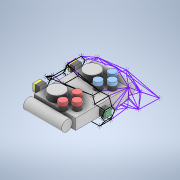
# Autodesk Inventor part: Obudowa_v1
Saved by Autodesk Inventor 2020 (Build 240168000, 168)
## iProperties
Created: 2020-04-14
Part Number: Obudowa_v1
Material: Generic
Document SubType Name: Modeling
Designer: atmat
Density: 1 g/cm^3
Appearance: Default
Author: atmat
Autodesk Inventor part; units mm, degrees
ref_plane "XY Plane" through (0, 0, 0) normal (0, 0, 1) x (1, 0, 0)
sketch "Sketch1" plane through (0, 0, 0) normal (0, 1, 0) x (-1, 0, 0)
  line L0 (35.245, 45.085) -> (-35.245, 45.085)
  line L1 (-35.245, 45.085) -> (-35.245, -45.085)
  line L2 (-35.245, -45.085) -> (35.245, -45.085)
  line L3 (35.245, -45.085) -> (35.245, 45.085)
  circle A0 centre (11.745, 29.845) radius 13
  circle A1 centre (11.745, -29.845) radius 13
  line L4 (-10.475, 45.085) -> (-10.475, -45.085) construction
  circle A2 centre (-10.475, 41.905) radius 6.5
  circle A3 centre (-10.475, 17.775) radius 6.5
  circle A4 centre (-10.475, -17.775) radius 6.5
  circle A5 centre (-10.475, -41.905) radius 6.5
  circle A6 centre (-22.545, 29.845) radius 6.5
  circle A7 centre (-22.545, -29.845) radius 6.5
  point P0 (0, 0)
  dimension "d0" = 90.17
  dimension "d1" = 45.085
  dimension "d2" = 35.245
  dimension "d3" = 70.49
  dimension "d4" = 15.24
  dimension "d5" = 15.24
  dimension "d6" = 23.5
  dimension "d7" = 23.5
  dimension "d8" = 26
  dimension "d9" = 26
  dimension "d10" = 45.72
  dimension "d11" = 13
  dimension "d12" = 13
  dimension "d13" = 13
  dimension "d14" = 13
  dimension "d15" = 3.18
  dimension "d16" = 3.18
  dimension "d17" = 24.13
  dimension "d18" = 24.13
  dimension "d19" = 13
  dimension "d20" = 12.07
  dimension "d21" = 12.07
  dimension "d22" = 0
  dimension "d23" = 0
  dimension "d24" = 13
  constraints: 10 end point, 8 centre point, 6 point on line, 2 parallel, 2 perpendicular, 1 horizontal
  measures "d0" distance of L2.end L0.start
  measures "d1" distance from line of point (0, 0) L0
  measures "d2" distance from line of point (0, 0) L3
  measures "d3" distance of L1.end L2.end
  measures "d4" distance from line of L0 A0.centre
  measures "d5" distance from line of L2 A1.centre
  measures "d6" distance from line of L3 A1.centre
  measures "d7" distance from line of L3 A0.centre
  measures "d8" diameter of A0
  measures "d9" diameter of A1
  measures "d10" distance between parallel lines of L3 L4
  measures "d11" diameter of A2
  measures "d12" diameter of A3
  measures "d13" diameter of A4
  measures "d14" diameter of A5
  measures "d15" distance from line of L0 A2.centre
  measures "d16" distance from line of L2 A5.centre
  measures "d17" distance of A3.centre A2.centre
  measures "d18" distance of A4.centre A5.centre
  measures "d19" diameter of A6
  measures "d20" horizontal distance of A2.centre A6.centre
  measures "d21" horizontal distance of A5.centre A7.centre
  measures "d22" vertical distance of A6.centre A0.centre
  measures "d23" vertical distance of A7.centre A1.centre
  measures "d24" diameter of A7
extrude "Extrusion1" add sketch "Sketch1" along normal blind 11 contours A0 | A1
sketch "Sketch2" plane through (0, 0, 0) normal (0, 1, 0) x (-1, 0, 0)
  line L0 (35.245, 45.085) -> (-35.245, 45.085)
  line L1 (-35.245, 45.085) -> (-35.245, -45.085)
  line L2 (-35.245, -45.085) -> (35.245, -45.085)
  line L3 (35.245, -45.085) -> (35.245, 45.085)
  circle A0 centre (11.745, 29.845) radius 13
  circle A1 centre (11.745, -29.845) radius 13
  line L4 (-10.475, 45.085) -> (-10.475, -45.085) construction
  circle A2 centre (-10.475, 41.905) radius 6.5
  circle A3 centre (-10.475, 17.775) radius 6.5
  circle A4 centre (-10.475, -17.775) radius 6.5
  circle A5 centre (-10.475, -41.905) radius 6.5
  circle A6 centre (-22.545, 29.845) radius 6.5
  circle A7 centre (-22.545, -29.845) radius 6.5
  point P0 (0, 0)
  dimension "d27" = 90.17
  dimension "d28" = 45.085
  dimension "d29" = 35.245
  dimension "d30" = 70.49
  dimension "d31" = 15.24
  dimension "d32" = 15.24
  dimension "d33" = 23.5
  dimension "d34" = 23.5
  dimension "d35" = 26
  dimension "d36" = 26
  dimension "d37" = 45.72
  dimension "d38" = 13
  dimension "d39" = 13
  dimension "d40" = 13
  dimension "d41" = 13
  dimension "d42" = 3.18
  dimension "d43" = 3.18
  dimension "d44" = 24.13
  dimension "d45" = 24.13
  dimension "d46" = 13
  dimension "d47" = 12.07
  dimension "d48" = 12.07
  dimension "d49" = 0
  dimension "d50" = 0
  dimension "d51" = 13
  constraints: 10 end point, 8 centre point, 6 point on line, 2 parallel, 2 perpendicular, 1 horizontal
  measures "d27" distance of L2.end L0.start
  measures "d28" distance from line of point (0, 0) L0
  measures "d29" distance from line of point (0, 0) L3
  measures "d30" distance of L1.end L2.end
  measures "d31" distance from line of L0 A0.centre
  measures "d32" distance from line of L2 A1.centre
  measures "d33" distance from line of L3 A1.centre
  measures "d34" distance from line of L3 A0.centre
  measures "d35" diameter of A0
  measures "d36" diameter of A1
  measures "d37" distance between parallel lines of L3 L4
  measures "d38" diameter of A2
  measures "d39" diameter of A3
  measures "d40" diameter of A4
  measures "d41" diameter of A5
  measures "d42" distance from line of L0 A2.centre
  measures "d43" distance from line of L2 A5.centre
  measures "d44" distance of A3.centre A2.centre
  measures "d45" distance of A4.centre A5.centre
  measures "d46" diameter of A6
  measures "d47" horizontal distance of A2.centre A6.centre
  measures "d48" horizontal distance of A5.centre A7.centre
  measures "d49" vertical distance of A6.centre A0.centre
  measures "d50" vertical distance of A7.centre A1.centre
  measures "d51" diameter of A7
extrude "Extrusion2" add sketch "Sketch2" along normal blind 7 contours A2 L0 | L0 A2 | A5 L2 | L2 A5 | A3 | A4 | A6 | A7
ref_plane "Work Plane1" through (0, 7, 0) normal (0, 1, 0) x (-1, 0, 0)
sketch "Sketch3" plane through (0, 7, 0) normal (0, 1, 0) x (-1, 0, 0)
  line L0 (35.245, 45.085) -> (-35.245, 45.085)
  line L1 (-35.245, 45.085) -> (-35.245, -45.085)
  line L2 (-35.245, -45.085) -> (35.245, -45.085)
  line L3 (35.245, -45.085) -> (35.245, 45.085)
  circle A0 centre (11.745, 29.845) radius 13
  circle A1 centre (11.745, -29.845) radius 13
  line L4 (-10.475, 45.085) -> (-10.475, -45.085) construction
  circle A2 centre (-10.475, 41.905) radius 6.5
  circle A3 centre (-10.475, 17.775) radius 6.5
  circle A4 centre (-10.475, -17.775) radius 6.5
  circle A5 centre (-10.475, -41.905) radius 6.5
  circle A6 centre (-22.545, 29.845) radius 6.5
  circle A7 centre (-22.545, -29.845) radius 6.5
  point P0 (0, 0)
  dimension "d55" = 90.17
  dimension "d56" = 45.085
  dimension "d57" = 35.245
  dimension "d58" = 70.49
  dimension "d59" = 15.24
  dimension "d60" = 15.24
  dimension "d61" = 23.5
  dimension "d62" = 23.5
  dimension "d63" = 26
  dimension "d64" = 26
  dimension "d65" = 45.72
  dimension "d66" = 13
  dimension "d67" = 13
  dimension "d68" = 13
  dimension "d69" = 13
  dimension "d70" = 3.18
  dimension "d71" = 3.18
  dimension "d72" = 24.13
  dimension "d73" = 24.13
  dimension "d74" = 13
  dimension "d75" = 12.07
  dimension "d76" = 12.07
  dimension "d77" = 0
  dimension "d78" = 0
  dimension "d79" = 13
  constraints: 10 end point, 8 centre point, 6 point on line, 2 parallel, 2 perpendicular, 1 horizontal
  measures "d55" distance of L2.end L0.start
  measures "d56" distance from line of point (0, 0) L0
  measures "d57" distance from line of point (0, 0) L3
  measures "d58" distance of L1.end L2.end
  measures "d59" distance from line of L0 A0.centre
  measures "d60" distance from line of L2 A1.centre
  measures "d61" distance from line of L3 A1.centre
  measures "d62" distance from line of L3 A0.centre
  measures "d63" diameter of A0
  measures "d64" diameter of A1
  measures "d65" distance between parallel lines of L3 L4
  measures "d66" diameter of A2
  measures "d67" diameter of A3
  measures "d68" diameter of A4
  measures "d69" diameter of A5
  measures "d70" distance from line of L0 A2.centre
  measures "d71" distance from line of L2 A5.centre
  measures "d72" distance of A3.centre A2.centre
  measures "d73" distance of A4.centre A5.centre
  measures "d74" diameter of A6
  measures "d75" horizontal distance of A2.centre A6.centre
  measures "d76" horizontal distance of A5.centre A7.centre
  measures "d77" vertical distance of A6.centre A0.centre
  measures "d78" vertical distance of A7.centre A1.centre
  measures "d79" diameter of A7
extrude "Extrusion3" add sketch "Sketch3" along normal blind 6 separate body contours A2 L0 | L0 A2 | A5 L2 | L2 A5 | A3 | A4 | A6 | A7
sketch "Sketch4" plane through (0, 0, 0) normal (0, 1, 0) x (-1, 0, 0)
  line L0 (35.245, 45.085) -> (-35.245, 45.085)
  line L1 (-35.245, 45.085) -> (-35.245, -45.085)
  line L2 (-35.245, -45.085) -> (35.245, -45.085)
  line L3 (35.245, -45.085) -> (35.245, 45.085)
  circle A0 centre (11.745, 29.845) radius 13
  circle A1 centre (11.745, -29.845) radius 13
  line L4 (-10.475, 45.085) -> (-10.475, -45.085) construction
  circle A2 centre (-10.475, 41.905) radius 6.5
  circle A3 centre (-10.475, 17.775) radius 6.5
  circle A4 centre (-10.475, -17.775) radius 6.5
  circle A5 centre (-10.475, -41.905) radius 6.5
  circle A6 centre (-22.545, 29.845) radius 6.5
  circle A7 centre (-22.545, -29.845) radius 6.5
  point P0 (0, 0)
  dimension "d82" = 90.17
  dimension "d83" = 45.085
  dimension "d84" = 35.245
  dimension "d85" = 70.49
  dimension "d86" = 15.24
  dimension "d87" = 15.24
  dimension "d88" = 23.5
  dimension "d89" = 23.5
  dimension "d90" = 26
  dimension "d91" = 26
  dimension "d92" = 45.72
  dimension "d93" = 13
  dimension "d94" = 13
  dimension "d95" = 13
  dimension "d96" = 13
  dimension "d97" = 3.18
  dimension "d98" = 3.18
  dimension "d99" = 24.13
  dimension "d100" = 24.13
  dimension "d101" = 13
  dimension "d102" = 12.07
  dimension "d103" = 12.07
  dimension "d104" = 0
  dimension "d105" = 0
  dimension "d106" = 13
  constraints: 10 end point, 8 centre point, 6 point on line, 2 parallel, 2 perpendicular, 1 horizontal
  measures "d82" distance of L2.end L0.start
  measures "d83" distance from line of point (0, 0) L0
  measures "d84" distance from line of point (0, 0) L3
  measures "d85" distance of L1.end L2.end
  measures "d86" distance from line of L0 A0.centre
  measures "d87" distance from line of L2 A1.centre
  measures "d88" distance from line of L3 A1.centre
  measures "d89" distance from line of L3 A0.centre
  measures "d90" diameter of A0
  measures "d91" diameter of A1
  measures "d92" distance between parallel lines of L3 L4
  measures "d93" diameter of A2
  measures "d94" diameter of A3
  measures "d95" diameter of A4
  measures "d96" diameter of A5
  measures "d97" distance from line of L0 A2.centre
  measures "d98" distance from line of L2 A5.centre
  measures "d99" distance of A3.centre A2.centre
  measures "d100" distance of A4.centre A5.centre
  measures "d101" diameter of A6
  measures "d102" horizontal distance of A2.centre A6.centre
  measures "d103" horizontal distance of A5.centre A7.centre
  measures "d104" vertical distance of A6.centre A0.centre
  measures "d105" vertical distance of A7.centre A1.centre
  measures "d106" diameter of A7
extrude "Extrusion4" add sketch "Sketch4" against normal blind 18 contours L3 L2 A5 L1 L0 A2 | A2 L0 | L2 A5 | A0 | A1 | A3 | A4 | A6 | A7 picked at (-10.0855, 41.5356) picked at (-10.2378, -41.8714) bodies 1
ref_plane "Work Plane2" through (-35.245, 0, 0) normal (1, 0, 0) x (0, 1, 0)
sketch "Sketch6" plane through (-35.245, 0, 0) normal (1, 0, 0) x (0, 1, 0)
  circle A0 centre (0, -29.845) radius 6.5
  circle A1 centre (0, 29.845) radius 6.5
  line L0 (0, -45.085) -> (0, 45.085) projected
  line L1 (6, -23.845) -> (-6, -23.845)
  line L2 (-6, -23.845) -> (-6, -35.845)
  line L3 (-6, -35.845) -> (6, -35.845)
  line L4 (6, -35.845) -> (6, -23.845)
  line L5 (6, 35.845) -> (-6, 35.845)
  line L6 (-6, 35.845) -> (-6, 23.845)
  line L7 (-6, 23.845) -> (6, 23.845)
  line L8 (6, 23.845) -> (6, 35.845)
  point P0 (0, 0)
  dimension "d114" = 13
  dimension "d115" = 13
  dimension "d116" = 59.69
  dimension "d117" = 29.845
  dimension "d149" = 12
  dimension "d150" = 12
  dimension "d151" = 6
  dimension "d152" = 6
  dimension "d153" = 12
  dimension "d154" = 12
  dimension "d155" = 6
  dimension "d156" = 6
  constraints: 16 end point, 4 parallel, 2 centre point, 2 horizontal, 2 perpendicular, 2 point on line
  measures "d114" diameter of A0
  measures "d115" diameter of A1
  measures "d116" distance of A1.centre A0.centre
  measures "d117" distance of point (0, 0) A0.centre
  measures "d149" distance of L5.start L5.end
  measures "d150" distance of L5.end L6.end
  measures "d151" distance from line of A1.centre L5
  measures "d152" distance from line of L6 A1.centre
  measures "d153" distance of L1.start L1.end
  measures "d154" distance of L1.end L2.end
  measures "d155" distance from line of A0.centre L1
  measures "d156" distance from line of A0.centre L2
extrude "Extrusion5" add sketch "Sketch6" against normal blind 7 contours L4 A0 L3 L0 L1 | A0 L1 L4 | L4 L3 A0 | L0 L3 A0 L2 L1 | A0 L2 L1 | L3 L2 A0 | L8 A1 L7 L0 L5 | A1 L5 L8 | L8 L7 A1 | L0 L7 A1 L6 L5 | A1 L6 L5 | L7 L6 A1 bodies 1
ref_plane "Work Plane3" through (-42.245, 0, 0) normal (1, 0, 0) x (0, 1, 0)
sketch "Sketch8" plane through (-35.245, 0, 0) normal (1, 0, 0) x (0, 1, 0)
  circle A0 centre (-9, 54.085) radius 9
  circle A1 centre (-9, -54.085) radius 9
  line L0 (0, 45.085) -> (-18, 45.085) projected
  line L1 (0, -45.085) -> (-18, -45.085) projected
  point P0 (0, 0)
  dimension "d127" = 18
  dimension "d128" = 18
  dimension "d129" = 9
  dimension "d130" = 9
  constraints: 2 centre point, 2 tangent
  measures "d127" diameter of A0
  measures "d128" diameter of A1
  measures "d129" horizontal distance of A1.centre point (0, 0)
  measures "d130" horizontal distance of A0.centre point (0, 0)
extrude "Extrusion7" add sketch "Sketch8" along normal blind 65 separate body
sketch "Sketch9" plane through (0, 7, 0) normal (0, 1, 0) x (-1, 0, 0)
  line L0 (25.245, 13.5) -> (-1.755, 13.5)
  line L1 (-1.755, 13.5) -> (-1.755, -13.5)
  line L2 (-1.755, -13.5) -> (25.245, -13.5)
  line L3 (25.245, -13.5) -> (25.245, 13.5)
  circle A0 centre (11.745, 29.845) radius 13 projected
  circle A1 centre (11.745, 29.845) radius 13
  point P0 (0, 0)
  dimension "d133" = 27
  dimension "d134" = 27
  dimension "d135" = 13.5
  dimension "d136" = 13.5
  constraints: 8 end point, 2 parallel, 1 centre point, 1 coincident, 1 horizontal, 1 perpendicular
  measures "d133" distance of L2.end L0.start
  measures "d134" distance of L1.end L2.end
  measures "d135" distance from line of point (0, 0) L2
  measures "d136" distance from line of L3 A1.centre
sketch "Sketch10" plane through (35.245, 0, 45.085) normal (1, 0, 0) x (0, 0, -1)
  line L0 (40.085, -16) -> (50.085, -16)
  line L1 (50.085, -16) -> (50.085, -6)
  line L2 (50.085, -6) -> (40.085, -6)
  line L3 (40.085, -6) -> (40.085, -16)
  line L4 (0, 0) -> (90.17, 0) projected
  point P0 (45.085, 0)
  dimension "d137" = 10
  dimension "d138" = 10
  dimension "d140" = 5
  dimension "d171" = 6
  constraints: 8 end point, 2 parallel, 1 horizontal, 1 perpendicular
  measures "d137" distance of L1.end L2.end
  measures "d138" distance of L0.end L1.end
  measures "d140" distance from line of point (45.085, 0) L1
  measures "d171" distance between parallel lines of L4 L2
extrude "Extrusion8" add sketch "Sketch10" along normal blind 7 bodies 1
sketch "Sketch11" plane through (42.245, 0, 45.085) normal (1, 0, 0) x (0, 0, -1)
  line L0 (40.085, -16) -> (50.085, -16)
  line L1 (50.085, -16) -> (50.085, -6)
  line L2 (50.085, -6) -> (40.085, -6)
  line L3 (40.085, -6) -> (40.085, -16)
  line L4 (0, 0) -> (90.17, 0) projected
  point P0 (45.085, 0)
  dimension "d143" = 10
  dimension "d144" = 10
  dimension "d146" = 5
  dimension "d172" = 6
  constraints: 8 end point, 2 parallel, 1 horizontal, 1 perpendicular
  measures "d143" distance of L1.end L2.end
  measures "d144" distance of L0.end L1.end
  measures "d146" distance from line of point (45.085, 0) L1
  measures "d172" distance between parallel lines of L4 L2
extrude "Extrusion9" add sketch "Sketch11" along normal blind 3 separate body
sketch "Sketch12" plane through (-42.245, 0, 0) normal (1, 0, 0) x (0, 1, 0)
  circle A0 centre (0, -29.845) radius 6.5
  circle A1 centre (0, 29.845) radius 6.5
  line L0 (6, -23.845) -> (-6, -23.845)
  line L1 (-6, -23.845) -> (-6, -35.845)
  line L2 (-6, -35.845) -> (6, -35.845)
  line L3 (6, -35.845) -> (6, -23.845)
  line L4 (6, 35.845) -> (-6, 35.845)
  line L5 (-6, 35.845) -> (-6, 23.845)
  line L6 (-6, 23.845) -> (6, 23.845)
  line L7 (6, 23.845) -> (6, 35.845)
  point P0 (0, 0)
  dimension "d157" = 13
  dimension "d158" = 13
  dimension "d159" = 59.69
  dimension "d160" = 29.845
  dimension "d161" = 12
  dimension "d162" = 12
  dimension "d163" = 6
  dimension "d164" = 6
  dimension "d165" = 12
  dimension "d166" = 12
  dimension "d167" = 6
  dimension "d168" = 6
  constraints: 16 end point, 4 parallel, 2 centre point, 2 horizontal, 2 perpendicular
  measures "d157" diameter of A0
  measures "d158" diameter of A1
  measures "d159" distance of A1.centre A0.centre
  measures "d160" distance of point (0, 0) A0.centre
  measures "d161" distance of L4.start L4.end
  measures "d162" distance of L4.end L5.end
  measures "d163" distance from line of A1.centre L4
  measures "d164" distance from line of L5 A1.centre
  measures "d165" distance of L0.start L0.end
  measures "d166" distance of L0.end L1.end
  measures "d167" distance from line of A0.centre L0
  measures "d168" distance from line of A0.centre L1
extrude "Extrusion10" add sketch "Sketch12" against normal blind 4 separate body contours L3 A0 L2 L1 L0 | A0 L0 L3 | L3 L2 A0 | A0 L1 L0 | L2 L1 A0 | L7 A1 L6 L5 L4 | A1 L4 L7 | L7 L6 A1 | A1 L5 L4 | L6 L5 A1
sketch3d "3D Sketch1"
body "Solid1"
body "Solid2"
body "Solid4"
body "Solid5"
body "Solid6"
